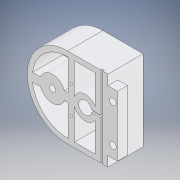
# Autodesk Inventor part: AA005b
Saved by Autodesk Inventor 2017 SP1 (Build 210196100, 196)
## iProperties
Created: 2017-06-04
Part Number: AA005b
Material: ABS Plastic
Document SubType Name: Modeling
Designer: Zach
Density: 1.06 g/cm^3
Appearance: CR White
Author: Zach
Autodesk Inventor part; units mm, degrees
ref_plane "YZ Plane" through (0, 0, 0) normal (1, 0, 0) x (0, 1, 0)
ref_plane "XZ Plane" through (0, 0, 0) normal (0, 1, 0) x (-1, 0, 0)
ref_plane "XY Plane" through (0, 0, 0) normal (0, 0, 1) x (1, 0, 0)
sketch "Sketch1" plane through (0, 0, 0) normal (0, 0, 1) x (1, 0, 0)
  line L0 (0, 0) -> (160, 0)
  line L1 (160, 0) -> (160, 160)
  line L2 (160, 160) -> (0, 160)
  line L3 (0, 160) -> (0, 0)
  circle A0 centre (50, 80) radius 6
  point P0 (160, 80)
  dimension "d0" = 160
  dimension "d1" = 160
  dimension "d2" = 12
  dimension "d7" = 50
  constraints: 8 end point, 2 parallel, 1 centre point, 1 horizontal, 1 horizontal alignment, 1 midpoint, 1 perpendicular
  measures "d0" distance of L2.end L1.end
  measures "d1" distance of L1.end L0.end
  measures "d2" diameter of A0
  measures "d7" distance from line of L3 A0.centre
extrude "Extrusion1" add sketch "Sketch1" along normal blind 70
sketch "Sketch2" plane through (0, 0, 70) normal (0, 0, 1) x (1, 0, 0)
  circle A0 centre (115, 80) radius 2.5
  line L0 (160, 0) -> (160, 160) projected
  circle A1 centre (50, 80) radius 6 projected
  line L1 (0, 0) -> (160, 0) projected
  line L2 (160, 0) -> (160, 160) projected
  line L3 (160, 160) -> (0, 160) projected
  line L4 (0, 160) -> (0, 0) projected
  point P0 (160, 80)
  dimension "d8" = 5
  dimension "d9" = 65
  constraints: 1 centre point, 1 horizontal alignment, 1 midpoint
  measures "d8" diameter of A0
  measures "d9" distance of A0.centre A1.centre
extrude "Extrusion2" cut sketch "Sketch2" against normal through all contours A0
sketch "Sketch5" plane through (0, 0, 70) normal (0, 0, 1) x (1, 0, 0)
  circle A0 centre (50, 80) radius 6 projected
  line L0 (0, 0) -> (160, 0) projected
  line L1 (160, 0) -> (160, 160) projected
  line L2 (160, 160) -> (0, 160) projected
  line L3 (0, 160) -> (0, 0) projected
  circle A1 centre (80, 80) radius 80 construction
  line L4 (0, 0) -> (160, 0) projected
  arc A2 (80, 160) -> (80, 0) centre (80, 80) ccw
  line L5 (160, 160) -> (0, 160) projected
  line L6 (80, 160) -> (0, 160)
  line L7 (0, 160) -> (0, 0)
  line L8 (80, 0) -> (0, 0)
  point P0 (0, 80)
  constraints: 6 end point, 4 point on circle, 4 tangent, 3 midpoint, 2 centre point, 2 collinear, 1 horizontal alignment, 1 perpendicular
extrude "Extrusion5" cut sketch "Sketch5" against normal through all contours L3 A2 L0 | L3 L2 A2
sketch "Sketch21" plane through (0, 0, 70) normal (0, 0, 1) x (1, 0, 0)
  circle A0 centre (115, 80) radius 2.5 projected
  circle A1 centre (115, 80) radius 13
  point P0 (0, 0)
  dimension "d100" = 26
  constraints: 1 centre point, 1 coincident
  measures "d100" diameter of A1
extrude "Extrusion21" cut sketch "Sketch21" against normal blind 65
sketch "Sketch22" plane through (115, 80, 5) normal (0, 0, 1) x (1, 0, 0)
  circle A0 centre (0, 8.5) radius 2
  circle A1 centre (0, -8.5) radius 2
  circle A2 centre (0, 0) radius 2.5 construction
  line L0 (0, 8.5) -> (0, -8.5) construction
  point P0 (-115, -80)
  dimension "d103" = 4
  dimension "d104" = 4
  dimension "d105" = 17
  constraints: 2 centre point, 2 end point, 2 vertical alignment, 1 coincident, 1 midpoint, 1 vertical
  measures "d103" diameter of A0
  measures "d104" diameter of A1
  measures "d105" distance of L0.start L0.end
extrude "Extrusion22" cut sketch "Sketch22" against normal through all
sketch "Sketch23" plane through (0, 0, 0) normal (0, 0, -1) x (-1, 0, 0)
  circle A0 centre (-115, 88.5) radius 2 projected
  circle A1 centre (-115, 71.5) radius 2 projected
  circle A2 centre (-115, 88.5) radius 3.5
  circle A3 centre (-115, 71.5) radius 3.5
  point P0 (0, 0)
  dimension "d108" = 7
  dimension "d109" = 7
  constraints: 2 centre point, 2 coincident
  measures "d108" diameter of A2
  measures "d109" diameter of A3
extrude "Extrusion23" cut sketch "Sketch23" against normal blind 3 contours A0 | A1 | A2 | A3
sketch "Sketch24" plane through (115, 80, 5) normal (0, 0, 1) x (1, 0, 0)
  circle A0 centre (0, 0) radius 2.5 projected
  circle A1 centre (0, 0) radius 4
  point P0 (-115, -80)
  dimension "d112" = 8
  constraints: 1 centre point, 1 coincident
  measures "d112" diameter of A1
extrude "Extrusion24" cut sketch "Sketch24" against normal blind 3
sketch "Sketch25" plane through (0, 0, 70) normal (0, 0, 1) x (1, 0, 0)
  line L0 (115, 77.5) -> (150, 77.5)
  line L1 (150, 77.5) -> (150, 82.5)
  line L2 (150, 82.5) -> (115, 82.5)
  line L3 (115, 82.5) -> (115, 77.5)
  line L4 (160, 0) -> (160, 160) projected
  line L5 (80, 0) -> (160, 0) projected
  line L6 (160, 160) -> (80, 160) projected
  line L7 (150, 0) -> (145, 0)
  line L8 (145, 0) -> (145, 160)
  line L9 (145, 160) -> (150, 160)
  line L10 (150, 160) -> (150, 0)
  point P0 (0, 0)
  point P1 (115, 88.5)
  point P2 (150, 80)
  point P3 (160, 80)
  dimension "d115" = 10
  dimension "d116" = 5
  dimension "d119" = 5
  constraints: 16 end point, 4 parallel, 3 midpoint, 2 horizontal, 2 perpendicular, 2 point on line, 1 horizontal alignment, 1 vertical alignment
  measures "d115" distance between parallel lines of L4 L1
  measures "d116" distance of L8.end L9.end
  measures "d119" distance between parallel lines of L2 L0
extrude "Extrusion25" cut sketch "Sketch25" against normal blind 3 contours L3 L2 L8 L0 | L8 L2 L1 L0 | L0 L10 L5 L8 | L8 L6 L10 L2
sketch "Sketch26" plane through (0, 0, 70) normal (0, 0, 1) x (1, 0, 0)
  line L0 (160, 0) -> (160, 160) projected
  line L1 (160, 20) -> (179, 20)
  line L2 (179, 20) -> (179, 140)
  line L3 (179, 140) -> (160, 140)
  line L4 (160, 140) -> (160, 20)
  line L5 (80, 0) -> (145, 0) projected
  line L6 (145, 160) -> (80, 160) projected
  circle A0 centre (170, 42.5) radius 2.5
  line L7 (170, 117.5) -> (170, 42.5) construction
  circle A1 centre (170, 117.5) radius 2.5
  point P0 (0, 0)
  point P1 (179, 80)
  point P2 (170, 80)
  dimension "d120" = 19
  dimension "d121" = 20
  dimension "d122" = 20
  dimension "d123" = 5
  dimension "d124" = 10
  dimension "d142" = 75
  dimension "d143" = 5
  constraints: 10 end point, 2 centre point, 2 coincident, 2 midpoint, 2 parallel, 1 horizontal, 1 horizontal alignment, 1 perpendicular, 1 point on line, 1 vertical alignment
  measures "d120" distance of L3.end L2.end
  measures "d121" distance between parallel lines of L5 L1
  measures "d122" distance between parallel lines of L6 L3
  measures "d123" diameter of A0
  measures "d124" distance from line of L0 A0.centre
  measures "d142" distance of L7.start L7.end
  measures "d143" diameter of A1
extrude "Extrusion26" add sketch "Sketch26" against normal blind 20
sketch "Sketch27" plane through (0, 0, 70) normal (0, 0, 1) x (1, 0, 0)
  line L0 (179, 52.5) -> (87.5, 52.5) construction
  line L1 (87.5, 52.5) -> (87.5, 107.5) construction
  line L2 (87.5, 107.5) -> (179, 107.5) construction
  line L3 (179, 107.5) -> (179, 52.5) construction
  line L4 (179, 20) -> (179, 140) construction
  circle A0 centre (87.5, 52.5) radius 2.5
  circle A1 centre (87.5, 107.5) radius 2.5
  point P0 (0, 0)
  point P1 (179, 80)
  dimension "d127" = 91.5
  dimension "d128" = 55
  dimension "d129" = 5
  dimension "d130" = 5
  constraints: 8 end point, 2 centre point, 2 coincident, 2 midpoint, 2 parallel, 1 horizontal, 1 perpendicular
  measures "d127" distance of L1.end L2.end
  measures "d128" distance of L0.end L1.end
  measures "d129" diameter of A0
  measures "d130" diameter of A1
extrude "Extrusion27" cut sketch "Sketch27" against normal blind 25
sketch "Sketch28" plane through (0, 0, 0) normal (0, 0, -1) x (-1, 0, 0)
  circle A0 centre (-50, 80) radius 25
  circle A1 centre (-50, 80) radius 6 projected
  point P0 (0, 0)
  dimension "d133" = 50
  constraints: 1 centre point, 1 coincident
  measures "d133" diameter of A0
extrude "Extrusion28" cut sketch "Sketch28" against normal blind 6 contours A0 | A1
sketch "Sketch29" plane through (0, 0, 70) normal (0, 0, 1) x (1, 0, 0)
  circle A0 centre (170, 42.5) radius 2.5 projected
  circle A1 centre (170, 42.5) radius 6.5
  circle A2 centre (170, 117.5) radius 2.5 projected
  circle A3 centre (170, 117.5) radius 6.5
  point P0 (0, 0)
  dimension "d136" = 13
  dimension "d144" = 13
  constraints: 2 centre point, 2 coincident
  measures "d136" diameter of A1
  measures "d144" diameter of A3
extrude "Extrusion29" cut sketch "Sketch29" against normal blind 15 contours A0 | A1 | A3
sketch "Sketch30" plane through (0, 0, 70) normal (0, 0, 1) x (1, 0, 0)
  circle A0 centre (87.5, 52.5) radius 2.5 projected
  circle A1 centre (87.5, 107.5) radius 2.5 projected
  line L0 (145, 82.5) -> (145, 160) projected
  line L1 (145, 160) -> (80, 160) projected
  arc A2 (80, 160) -> (80, 0) centre (80, 80) ccw projected
  line L2 (80, 0) -> (145, 0) projected
  line L3 (145, 0) -> (145, 77.5) projected
  line L4 (145, 77.5) -> (127.7574, 77.5) projected
  arc A3 (127.7574, 82.5) -> (127.7574, 77.5) centre (115, 80) ccw projected
  line L5 (127.7574, 82.5) -> (145, 82.5) projected
  circle A4 centre (50, 80) radius 6 construction
  circle A5 centre (50, 80) radius 25 construction
  circle A6 centre (115, 88.5) radius 3.5 projected
  circle A7 centre (115, 71.5) radius 3.5 projected
  arc A8 (80, 160) -> (80, 0) centre (80, 80) ccw projected
  line L6 (160, 160) -> (80, 160) projected
  line L7 (160, 0) -> (160, 160) projected
  line L8 (80, 0) -> (160, 0) projected
  circle A9 centre (115, 80) radius 2.5 projected
  arc A10 (80, 150) -> (80, 10) centre (80, 80) ccw construction
  line L9 (80, 150) -> (135, 150) construction
  line L10 (135, 150) -> (135, 92.5)
  line L11 (135, 92.5) -> (134.3067, 92.5)
  arc A11 (134.3067, 92.5) -> (134.3067, 67.5) centre (115, 80) ccw construction
  line L12 (134.3067, 67.5) -> (135, 67.5)
  line L13 (135, 67.5) -> (135, 10)
  line L14 (135, 10) -> (80, 10) construction
  line L15 (93.6283, 71.5) -> (10.518, 71.5) construction
  line L16 (93.6283, 88.5) -> (10.518, 88.5) construction
  arc A12 (80, 150) -> (10.518, 88.5) centre (80, 80) ccw
  arc A13 (10.518, 71.5) -> (80, 10) centre (80, 80) ccw
  arc A14 (134.3067, 92.5) -> (93.6283, 88.5) centre (115, 80) ccw
  arc A15 (93.6283, 71.5) -> (134.3067, 67.5) centre (115, 80) ccw
  line L17 (81.3717, 150) -> (81.3717, 10) construction
  line L18 (93.6283, 88.5) -> (93.6283, 150)
  line L19 (93.6283, 71.5) -> (93.6283, 10)
  line L20 (87.5, 52.5) -> (87.5, 107.5) construction
  line L21 (80, 150) -> (81.3717, 150)
  line L22 (80, 10) -> (81.3717, 10)
  line L23 (93.6283, 10) -> (135, 10)
  line L24 (93.6283, 150) -> (135, 150)
  line L25 (81.3717, 150) -> (81.3717, 88.5)
  line L26 (81.3717, 71.5) -> (81.3717, 10)
  line L27 (10.518, 71.5) -> (81.3717, 71.5) construction
  line L28 (10.518, 88.5) -> (81.3717, 88.5) construction
  line L29 (10.518, 88.5) -> (26.4894, 88.5)
  circle A16 centre (50, 80) radius 25 construction
  line L30 (10.518, 71.5) -> (26.4894, 71.5)
  line L31 (81.3717, 71.5) -> (73.5106, 71.5)
  line L32 (81.3717, 88.5) -> (73.5106, 88.5)
  arc A17 (73.5106, 88.5) -> (26.4894, 88.5) centre (50, 80) ccw
  arc A18 (26.4894, 71.5) -> (73.5106, 71.5) centre (50, 80) ccw
  point P0 (0, 0)
  dimension "d139" = 10
  constraints: 48 end point, 24 point on circle, 13 point on line, 8 centre point, 6 concentric, 5 collinear, 4 tangent, 2 horizontal, 2 horizontal alignment, 2 perpendicular, 2 vertical, 1 parallel, 8 other
  measures "d139" radial gap between concentric circles of A2 A10
extrude "Extrusion30" cut sketch "Sketch30" against normal blind 60 contours L10 L11 A14 L18 L24 | L12 L13 L23 L19 A15 | L21 L25 L32 A17 L29 A12 | L30 A18 L31 L26 L22 A13
body "Solid1"
